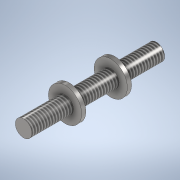
# Autodesk Inventor part: ось крепление пушки
Saved by Autodesk Inventor 2020.1 (Build 241239000, 239)
## iProperties
Created: 2022-03-19
Part Number: ось крепление пушки
Material: Железо, ковкое
Document SubType Name: Modeling
Designer: User
Density: 7.15 g/cm^3
Appearance: С умеренной полировкой
Author: User
Autodesk Inventor part; units mm, degrees
ref_plane "YZ Plane" through (0, 0, 0) normal (1, 0, 0) x (0, 1, 0)
ref_plane "XZ Plane" through (0, 0, 0) normal (0, 1, 0) x (-1, 0, 0)
ref_plane "XY Plane" through (0, 0, 0) normal (0, 0, 1) x (1, 0, 0)
sketch "Эскиз1" plane through (0, 0, 0) normal (0, 0, 1) x (1, 0, 0)
  circle A0 centre (0, 0) radius 2
  dimension "d0" = 4
  constraints: 1 centre point, 1 coincident
  measures "d0" diameter of A0
extrude "Выдавливание1" add sketch "Эскиз1" along normal blind 10
sketch "Эскиз2" plane through (0, 0, 10) normal (0, 0, 1) x (1, 0, 0)
  circle A0 centre (0, 0) radius 4
  dimension "d5" = 8
  constraints: 1 centre point, 1 coincident
  measures "d5" diameter of A0
extrude "Выдавливание2" add sketch "Эскиз2" along normal blind 0.5
mirror "Зеркальное отражение1" about plane through (0, 0, 10.5) normal (0, 0, 1) of "Выдавливание2", "Выдавливание1"
sketch "Эскиз3" plane through (0, 0, 21) normal (0, 0, 1) x (1, 0, 0)
  circle A0 centre (-7.3376, 4.7247) radius 20.8096
  point P0 (0, 0)
  constraints: 1 centre point
extrude "Выдавливание3" cut sketch "Эскиз3" against normal blind 5
mirror "Зеркальное отражение3" about plane through (-7.3376, 4.7247, 16) normal (0, 0, 1)
thread "Резьба4" size "M4x0.7" class "6g" standard "ANSI Metric M Profile" full length
